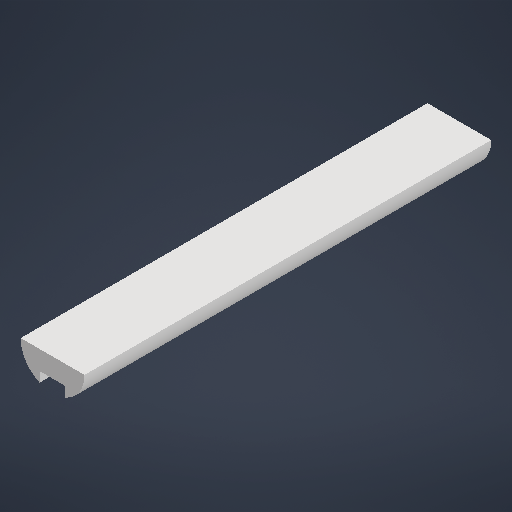
# Autodesk Inventor part: Long_axel
Saved by Autodesk Inventor 2026 (Build 300175050, 175E)
## iProperties
Created: 2026-05-01
Part Number: Long_axel
Material: Generic
Document SubType Name: Modeling
Designer: sniel
Density: 1 g/cm^3
Appearance: Default
Author: sniel
Autodesk Inventor part; units mm, degrees
ref_plane "YZ Plane" through (0, 0, 0) normal (1, 0, 0) x (0, 1, 0)
ref_plane "XZ Plane" through (0, 0, 0) normal (0, 1, 0) x (-1, 0, 0)
ref_plane "XY Plane" through (0, 0, 0) normal (0, 0, 1) x (1, 0, 0)
sketch "Sketch1" plane through (0, 0, 0) normal (0, 0, 1) x (1, 0, 0)
  line L0 (1.5575, -2.3616) -> (1.5482, -3.6067)
  line L1 (-1.5924, -2.3382) -> (1.5575, -2.3616)
  line L2 (-1.6017, -3.5833) -> (-1.5924, -2.3382)
  arc A0 (-1.5482, 3.6067) -> (-1.6017, -3.5833) centre (0, 0) ccw
  line L3 (-1.5575, 2.3616) -> (-1.5482, 3.6067)
  line L4 (1.5924, 2.3382) -> (-1.5575, 2.3616)
  line L5 (1.6017, 3.5833) -> (1.5924, 2.3382)
  arc A1 (1.5482, -3.6067) -> (1.6017, 3.5833) centre (0, 0) ccw
  point P0 (0, 0)
  constraints: 12 end point, 4 point on circle, 2 centre point
extrude "Extrusion1" add sketch "Sketch1" along normal blind 50
sketch "Sketch2" plane through (0, 0, 0) normal (0, 0, -1) x (-1, 0, 0)
  line L0 (-25, 13) -> (13, 13)
  line L1 (13, 13) -> (13, 0)
  line L2 (13, 0) -> (-25, 0)
  line L3 (-25, 0) -> (-25, 13)
  point P0 (0, 0)
  constraints: 8 end point, 2 parallel, 1 horizontal, 1 perpendicular
extrude "Extrusion2" cut sketch "Sketch2" against normal blind 89.5
body "Solid1"
